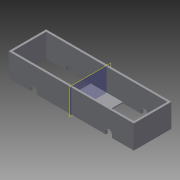
# Autodesk Inventor part: CarChassis
Saved by Autodesk Inventor 2015 (Build 190159000, 159)
## iProperties
Created: 2016-03-26
Part Number: CarChassis
Material: Generic
Document SubType Name: Modeling
Designer: Lee
Density: 1 g/cm^3
Appearance: Default
Author: Lee
Autodesk Inventor part; units mm, degrees
ref_plane "YZ Plane" through (0, 0, 0) normal (1, 0, 0) x (0, 1, 0)
ref_plane "XZ Plane" through (0, 0, 0) normal (0, 1, 0) x (-1, 0, 0)
ref_plane "XY Plane" through (0, 0, 0) normal (0, 0, 1) x (1, 0, 0)
sketch "Sketch1" plane through (0, 0, 0) normal (0, 0, 1) x (1, 0, 0)
  line L0 (0.8, -15.24) -> (-0.8, -15.24)
  line L1 (-0.8, -15.24) -> (-0.8, 15.24)
  line L2 (-0.8, 15.24) -> (0.8, 15.24)
  line L3 (0.8, 15.24) -> (0.8, -15.24)
  line L4 (0.8, -15.24) -> (-0.8, 15.24) construction
  line L5 (-0.8, -15.24) -> (0.8, 15.24) construction
  line L6 (-0.8, -15.24) -> (100.8, -15.24)
  line L7 (100.8, -15.24) -> (100.8, -13.64)
  line L8 (100.8, -13.64) -> (-0.8, -13.64)
  line L9 (-0.8, -13.64) -> (-0.8, -15.24)
  line L10 (-0.8, 15.24) -> (100.8, 15.24)
  line L11 (100.8, 15.24) -> (100.8, 13.64)
  line L12 (100.8, 13.64) -> (-0.8, 13.64)
  line L13 (-0.8, 13.64) -> (-0.8, 15.24)
  line L14 (100.8, -15.24) -> (99.2, -15.24)
  line L15 (99.2, -15.24) -> (99.2, 15.24)
  line L16 (99.2, 15.24) -> (100.8, 15.24)
  line L17 (100.8, 15.24) -> (100.8, -15.24)
  point P0 (0, 0)
  dimension "d0" = 1.6
  dimension "d1" = 30.48
  dimension "d2" = 101.6
  dimension "d3" = 1.6
  dimension "d4" = 101.6
  dimension "d5" = 1.6
  dimension "d6" = 1.6
  constraints: 36 end point, 8 parallel, 4 horizontal, 4 perpendicular, 2 midpoint, 1 point on line
  measures "d0" distance of L1.end L2.end
  measures "d1" distance of L0.end L1.end
  measures "d2" distance of L8.end L7.end
  measures "d3" distance of L7.end L6.end
  measures "d4" distance of L11.end L12.end
  measures "d5" distance of L10.end L11.end
  measures "d6" distance of L15.end L16.end
extrude "Extrusion1" add sketch "Sketch1" along normal blind 19.05 contours L0 L1 L8 L3 | L3 L8 L15 L6 | L8 L1 L12 L3 | L15 L8 L7 L6 | L12 L1 L2 L3 | L3 L10 L15 L12 | L15 L12 L17 L8 | L15 L10 L11 L12
sketch "Sketch2" plane through (-0.8, -15.24, 0) normal (0, -1, 0) x (1, 0, 0)
  line L0 (100, 0) -> (1.6, 0) projected
  line L1 (0, 0) -> (0, 19.05) projected
  line L2 (17.78, 0) -> (22.78, 0)
  line L3 (22.78, 0) -> (22.78, 2.4)
  line L4 (22.78, 2.4) -> (17.78, 2.4)
  line L5 (17.78, 2.4) -> (17.78, 0)
  arc A0 (22.78, 2.4) -> (17.78, 2.4) centre (20.28, 2.4) ccw
  point P0 (0.8, 0)
  dimension "d9" = 17.78
  dimension "d10" = 5
  dimension "d11" = 2.4
  constraints: 8 end point, 2 parallel, 2 point on circle, 2 tangent, 1 centre point, 1 horizontal, 1 perpendicular, 1 point on line
  measures "d9" distance from line of L1 L2.start
  measures "d10" distance of L4.end L3.end
  measures "d11" distance of L3.end L2.end
extrude "Extrusion2" cut sketch "Sketch2" against normal up to surface (30.48 mm away)
ref_plane "Work Plane1" through (50, -15.24, 0) normal (-1, 0, 0) x (0, 0, 1)
mirror "Mirror1" about plane through (50, -15.24, 0) normal (-1, 0, 0) of "Extrusion2"
sketch "Sketch4" plane through (-0.8, 15.24, 19.05) normal (0, 1, 0) x (1, 0, 0)
  line L0 (78.82, 19.05) -> (22.78, 19.05) projected
  line L1 (22.78, 19.05) -> (78.82, 19.05) projected
  line L2 (50.8, 19.05) -> (37.78, 19.05)
  line L3 (37.78, 19.05) -> (37.78, 18.25)
  line L4 (37.78, 18.25) -> (50.8, 18.25)
  line L5 (50.8, 18.25) -> (50.8, 19.05)
  line L6 (22.78, 19.05) -> (22.78, 16.65) projected
  line L7 (22.78, 19.05) -> (78.82, 19.05)
  line L8 (63.82, 19.05) -> (63.82, 18.25)
  line L9 (63.82, 18.25) -> (50.8, 18.25)
  line L10 (63.82, 19.05) -> (37.78, 19.05)
  line L11 (37.78, 19.05) -> (37.78, 18.25)
  line L12 (37.78, 18.25) -> (63.82, 18.25)
  line L13 (63.82, 18.25) -> (63.82, 19.05)
  point P0 (0.8, 19.05)
  dimension "d15" = 0.8
  dimension "d16" = 15
  constraints: 22 end point, 4 parallel, 4 symmetric about line, 2 horizontal, 2 perpendicular, 1 midpoint
  measures "d15" distance of L3.end L2.end
  measures "d16" distance between parallel lines of L6 L3
extrude "Extrusion3" add sketch "Sketch4" against normal up to surface (30.48 mm away)
body "Solid1"
